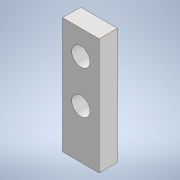
# Autodesk Inventor part: pcb_holder_3
Saved by Autodesk Inventor 2020 (Build 240168000, 168)
## iProperties
Created: 2019-07-23
Part Number: pcb_holder_3
Material: Generic
Document SubType Name: Modeling
Designer: psrob
Density: 1 g/cm^3
Appearance: Default
Author: psrob
Autodesk Inventor part; units mm, degrees
ref_plane "YZ Plane" through (0, 0, 0) normal (1, 0, 0) x (0, 1, 0)
ref_plane "XZ Plane" through (0, 0, 0) normal (0, 1, 0) x (-1, 0, 0)
ref_plane "XY Plane" through (0, 0, 0) normal (0, 0, 1) x (1, 0, 0)
sketch "Sketch1" plane through (0, 0, 0) normal (0, 0, 1) x (1, 0, 0)
  line L0 (32.6242, -2.1) -> (40.6242, -2.1) projected
  arc A0 (41.6242, -3.1) -> (40.6242, -2.1) centre (40.6242, -3.1) ccw projected
  line L1 (41.6242, -3.1) -> (41.6242, -14) projected
  line L2 (65.6275, -14) -> (41.6242, -14) projected
  line L3 (65.6275, -14) -> (65.6275, -2) projected
  arc A1 (67.6275, 0) -> (65.6275, -2) centre (67.6275, -2) ccw projected
  line L4 (67.6275, 0) -> (74, 0) projected
  line L5 (74, 0) -> (74, 2) projected
  line L6 (10, 2) -> (74, 2) projected
  line L7 (10, 2) -> (10, -14) projected
  line L8 (31.6242, -14) -> (10, -14) projected
  line L9 (31.6242, -14) -> (31.6242, -3.1) projected
  arc A2 (32.6242, -2.1) -> (31.6242, -3.1) centre (32.6242, -3.1) ccw projected
  circle A3 centre (12.5, -10.5) radius 1 projected
  circle A4 centre (59.6275, -9) radius 1.5 projected
  circle A5 centre (27.6275, -9) radius 1.5 projected
  circle A6 centre (17.6275, -2) radius 1.5 projected
  circle A7 centre (47.6275, -2) radius 1.5 projected
  circle A8 centre (59.6275, -2) radius 1.5 projected
  circle A9 centre (27.6275, -2) radius 1.5 projected
  circle A10 centre (17.6275, -9) radius 1.5 projected
  circle A11 centre (47.6275, -9) radius 1.5 projected
  line L10 (17.6275, -9) -> (17.6275, -2)
  line L11 (64.6275, -17) -> (10, -17) projected
  line L12 (20.6275, -13) -> (14.6275, -13)
  line L13 (14.6275, -13) -> (14.6275, 2)
  line L14 (14.6275, 2) -> (20.6275, 2)
  line L15 (20.6275, 2) -> (20.6275, -13)
  line L16 (20.6275, -13) -> (14.6275, 2) construction
  line L17 (14.6275, -13) -> (20.6275, 2) construction
  line L18 (20.6275, -13) -> (14.6275, -13)
  line L19 (14.6275, -13) -> (14.6275, -17)
  line L20 (14.6275, -17) -> (20.6275, -17)
  line L21 (20.6275, -17) -> (20.6275, -13)
  point P0 (0, 0)
  point P1 (17.6275, -5.5)
  dimension "d0" = 6
  dimension "d1" = 15
  dimension "d2" = 6
  dimension "d3" = 4
  constraints: 22 end point, 4 parallel, 3 midpoint, 3 perpendicular, 1 horizontal, 1 vertical
  measures "d0" distance of L12.start L12.end
  measures "d1" distance of L12.end L13.end
  measures "d2" distance of L20.end L19.end
  measures "d3" distance of L19.end L18.end
extrude "Extrusion1" add sketch "Sketch1" along normal blind 3 contours L21 L11 L19 L8 | L8 L19 L12 L21 | L12 L13 L6 L15
ref_plane "Work Plane1" through (-4, 0, -63) normal (0, 0, -1) x (-1, 0, 0)
sketch "Sketch2" plane through (-4, 0, -63) normal (0, 0, -1) x (-1, 0, 0)
  line L0 (32.6242, -2.1) -> (40.6242, -2.1) projected
  arc A0 (41.6242, -3.1) -> (40.6242, -2.1) centre (40.6242, -3.1) ccw projected
  line L1 (41.6242, -3.1) -> (41.6242, -14) projected
  line L2 (65.6275, -14) -> (41.6242, -14) projected
  line L3 (65.6275, -14) -> (65.6275, -2) projected
  arc A1 (67.6275, 0) -> (65.6275, -2) centre (67.6275, -2) ccw projected
  line L4 (67.6275, 0) -> (74, 0) projected
  line L5 (74, 0) -> (74, 2) projected
  line L6 (10, 2) -> (74, 2) projected
  line L7 (10, 2) -> (10, -14) projected
  line L8 (31.6242, -14) -> (10, -14) projected
  line L9 (31.6242, -14) -> (31.6242, -3.1) projected
  arc A2 (32.6242, -2.1) -> (31.6242, -3.1) centre (32.6242, -3.1) ccw projected
  circle A3 centre (12.5, -10.5) radius 1 projected
  circle A4 centre (59.6275, -9) radius 1.5 projected
  circle A5 centre (27.6275, -9) radius 1.5 projected
  circle A6 centre (17.6275, -2) radius 1.5 projected
  circle A7 centre (47.6275, -2) radius 1.5 projected
  circle A8 centre (59.6275, -2) radius 1.5 projected
  circle A9 centre (27.6275, -2) radius 1.5 projected
  circle A10 centre (17.6275, -9) radius 1.5 projected
  circle A11 centre (47.6275, -9) radius 1.5 projected
  line L10 (64.6275, -17) -> (10, -17) projected
  line L11 (17.6275, -9) -> (17.6275, -2)
  line L12 (14.6275, -13) -> (20.6275, -13)
  line L13 (20.6275, -13) -> (20.6275, 2)
  line L14 (20.6275, 2) -> (14.6275, 2)
  line L15 (14.6275, 2) -> (14.6275, -13)
  line L16 (14.6275, -13) -> (20.6275, 2) construction
  line L17 (20.6275, -13) -> (14.6275, 2) construction
  line L18 (14.6275, -13) -> (20.6275, -13)
  line L19 (20.6275, -13) -> (20.6275, -17)
  line L20 (20.6275, -17) -> (14.6275, -17)
  line L21 (14.6275, -17) -> (14.6275, -13)
  point P0 (-4, 0)
  point P1 (17.6275, -5.5)
  dimension "d6" = 6
  dimension "d7" = 15
  dimension "d8" = 6
  dimension "d9" = 4
  constraints: 22 end point, 4 parallel, 3 midpoint, 3 perpendicular, 1 horizontal, 1 vertical
  measures "d6" distance of L12.start L12.end
  measures "d7" distance of L13.end L12.end
  measures "d8" distance of L19.end L20.end
  measures "d9" distance of L18.end L19.end
extrude "Extrusion2" add sketch "Sketch2" along normal blind 3 contours L19 L10 L21 L8 | L8 L21 L12 L19 | L12 L15 L6 L13
sketch "Sketch3" plane through (-24.6275, -17, -63) normal (0, -1, 0) x (1, 0, 0)
  line L0 (6, 0) -> (0, 0) projected
  line L1 (0, 0) -> (0, -3) projected
  line L2 (6, -3) -> (0, -3) projected
  line L3 (6, 0) -> (6, -3) projected
  line L4 (39.255, 63) -> (45.255, 63) projected
  line L5 (45.255, 63) -> (45.255, 66) projected
  line L6 (39.255, 66) -> (45.255, 66) projected
  line L7 (39.255, 63) -> (39.255, 66) projected
  line L8 (45.255, 63) -> (6, -3)
  line L9 (39.255, 63) -> (39.255, 66) projected
  line L10 (39.255, 66) -> (0, 0)
  point P0 (24.6275, 63)
  constraints: 4 end point, 1 parallel
extrude "Extrusion3" add sketch "Sketch3" along normal blind 3
fillet "Fillet1" radius 1 2 edges at (14.6275, -17, 1.5) (-18.6275, -17, -64.5)
fillet "Fillet2" radius 2 4 edges at (-18.6275, 2, -64.5) (-24.6275, 2, -64.5) (20.6275, 2, 1.5) (14.6275, 2, 1.5)
body "Solid1"
